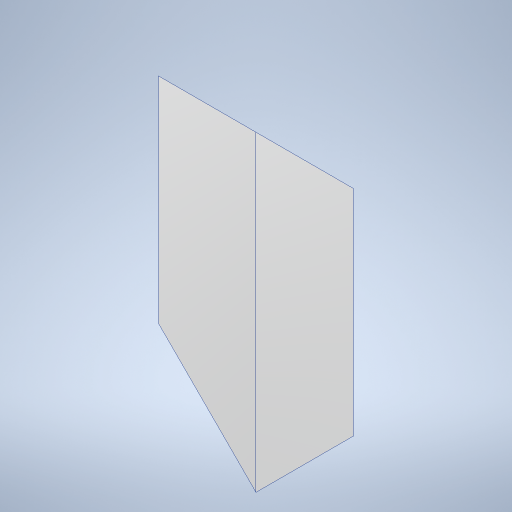
# Autodesk Inventor part: P404
Saved by Autodesk Inventor 2023 (Build 270158000, 158)
## iProperties
Created: 2022-08-29
Part Number: P404
Material: Aluminum 6061
Document SubType Name: Modeling
Designer: D.C. Eksteen
Density: 2.7 g/cm^3
Appearance: Aluminum - Flat
Author: D.C. Eksteen
Title: BRAKE REAR RISER
Autodesk Inventor part; units mm, degrees
ref_plane "YZ Plane" through (0, 0, 0) normal (1, 0, 0) x (0, 1, 0)
ref_plane "XZ Plane" through (0, 0, 0) normal (0, 1, 0) x (-1, 0, 0)
ref_plane "XY Plane" through (0, 0, 0) normal (0, 0, 1) x (1, 0, 0)
sketch "Sketch1" plane through (0, 0, 0) normal (0, 1, 0) x (-1, 0, 0)
  line L0 (0, 0) -> (25, 0)
  line L1 (25, 0) -> (25, -25)
  line L2 (25, -25) -> (0, -25)
  line L3 (0, -25) -> (0, 0)
  line L4 (22, -22) -> (22, -3)
  line L5 (22, -3) -> (3, -3)
  line L6 (3, -3) -> (3, -22)
  line L7 (3, -22) -> (22, -22)
  dimension "d0" = 25
  dimension "d1" = 25
  dimension "d2" = 3
  constraints: 16 end point, 4 parallel, 2 perpendicular, 1 horizontal, 3 other
  measures "d0" distance of L1.end L2.end
  measures "d1" distance of L0.end L1.end
  measures "d2" distance between parallel lines of L1 L4
extrude "Extrusion1" add sketch "Sketch1" along normal blind 80
sketch "Sketch2" plane through (0, 0, 0) normal (1, 0, 0) x (0, 0, -1)
  line L0 (0, 0) -> (25, 0) projected
  line L1 (25, 0) -> (25, 80) projected
  line L2 (0, 80) -> (25, 80) projected
  line L3 (0, 0) -> (0, 80) projected
  line L4 (0, 0) -> (0, 80) projected
  line L5 (0, 80) -> (25, 55)
  line L6 (0, 80) -> (35.3553, 80) construction
  dimension "d5" = 45
  constraints: 4 end point, 1 equal length, 1 horizontal, 1 point on line
  measures "d5" angle of L5 L6
extrude "Extrusion2" cut sketch "Sketch2" against normal blind 80 contours L2 L1 L5
sketch "Sketch3" plane through (-25, 0, 0) normal (0, 0, 1) x (1, 0, 0)
  line L0 (3, 0) -> (3, 77) projected
  line L1 (0, 0) -> (25, 0) projected
  line L2 (25, 0) -> (25, 80) projected
  line L3 (0, 80) -> (25, 80) projected
  line L4 (0, 0) -> (0, 80) projected
  line L5 (25, 0) -> (0, 0) projected
  line L6 (0, 25) -> (25, 0)
  dimension "d8" = 45
  constraints: 2 end point, 1 point on line
  measures "d8" angle of L1 L6
extrude "Extrusion3" cut sketch "Sketch3" against normal blind 44.75 contours L1 L4 L6 L0 | L0 L6 L1
body "Solid1"
